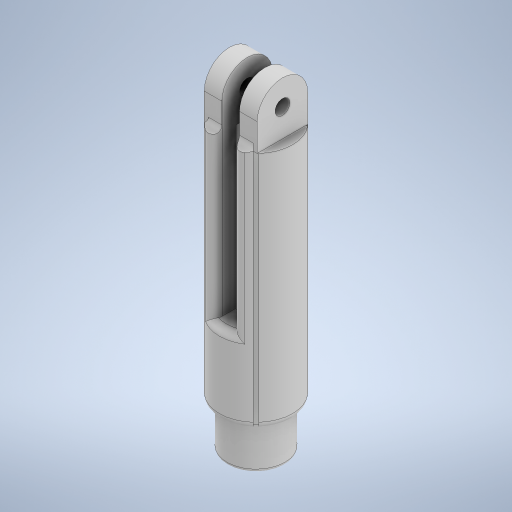
# Autodesk Inventor part: piston2
Saved by Autodesk Inventor 2024.2 (Build 282272000, 272)
## iProperties
Created: 2024-05-21
Part Number: piston2
Material: Generic
Document SubType Name: Modeling
Designer: Robin
Density: 1 g/cm^3
Appearance: Default
Author: Robin
Autodesk Inventor part; units mm, degrees
ref_plane "YZ Plane" through (0, 0, 0) normal (1, 0, 0) x (0, 1, 0)
ref_plane "XZ Plane" through (0, 0, 0) normal (0, 1, 0) x (-1, 0, 0)
ref_plane "XY Plane" through (0, 0, 0) normal (0, 0, 1) x (1, 0, 0)
sketch "Sketch1" plane through (0, 0, 0) normal (0, 1, 0) x (-1, 0, 0)
  circle A0 centre (0, 0) radius 10.375
  dimension "d0" = 20.75
  constraints: 1 centre point, 1 coincident
  measures "d0" diameter of A0
extrude "Extrusion1" add sketch "Sketch1" along normal blind 80
sketch "Sketch2" plane through (0, 80, 0) normal (0, 1, 0) x (1, 0, 0)
  line L0 (-10.375, -10.375) -> (10.375, -10.375)
  line L1 (10.375, -10.375) -> (10.375, 10.375)
  line L2 (10.375, 10.375) -> (-10.375, 10.375)
  line L3 (-10.375, 10.375) -> (-10.375, -10.375)
  circle A0 centre (0, 0) radius 10.375 projected
  line L4 (-2.5, -7.1687) -> (2.5, -7.1687)
  line L5 (2.5, -7.1687) -> (2.5, 7.1687)
  line L6 (2.5, 7.1687) -> (-2.5, 7.1687)
  line L7 (-2.5, 7.1687) -> (-2.5, -7.1687)
  line L8 (-10.375, -7.1687) -> (-7.5, -7.1687)
  line L9 (-7.5, -7.1687) -> (-7.5, 7.1687)
  line L10 (-7.5, 7.1687) -> (-10.375, 7.1687)
  line L11 (-10.375, 7.1687) -> (-10.375, -7.1687)
  line L12 (7.5, -7.1687) -> (10.375, -7.1687)
  line L13 (10.375, -7.1687) -> (10.375, 7.1687)
  line L14 (10.375, 7.1687) -> (7.5, 7.1687)
  line L15 (7.5, 7.1687) -> (7.5, -7.1687)
  line L16 (-7.5, -7.1687) -> (7.5, -7.1687)
  line L17 (-7.5, 7.1687) -> (7.5, 7.1687)
  point P0 (0, 7.1687)
  point P1 (2.5, 7.1687)
  point P2 (-2.5, 7.1687)
  dimension "d3" = 5
  dimension "d4" = 5
  dimension "d5" = 5
  constraints: 36 end point, 9 parallel, 5 horizontal, 4 perpendicular, 4 point on line, 4 tangent, 2 horizontal alignment, 2 point on circle, 1 midpoint, 1 vertical alignment
  measures "d3" distance between parallel lines of L5 L7
  measures "d4" distance between parallel lines of L9 L7
  measures "d5" distance between parallel lines of L5 L15
extrude "Extrusion2" add sketch "Sketch2" along normal blind 15 contours L9 L17 L7 L16 | L16 L5 L17 L15
sketch "Sketch4" plane through (0, 0, 0) normal (0, -1, 0) x (1, 0, 0)
  circle A0 centre (0, 0) radius 4
  line L0 (0, 0) -> (4, 0)
  line L1 (0, 0) -> (-2, -3.4641)
  line L2 (0, 0) -> (-2, 3.4641)
  circle A1 centre (0, 0) radius 10.375 projected
  line L3 (6.912, 7.7605) -> (7.7605, 6.912)
  line L4 (7.7605, 6.912) -> (6.3463, 5.4978)
  line L5 (6.3463, 5.4978) -> (5.4978, 6.3463)
  line L6 (5.4978, 6.3463) -> (6.912, 7.7605)
  line L7 (0, 0) -> (7.3362, 7.3362)
  line L8 (10.375, 0) -> (0, 0)
  point P0 (7.7482, 6.8997)
  point P1 (6.8997, 7.7482)
  dimension "d12" = 8
  dimension "d13" = 120
  dimension "d14" = 120
  dimension "d41" = 45
  dimension "d42" = 1.2
  dimension "d43" = 0.6
  dimension "d44" = 2
  constraints: 18 end point, 3 perpendicular, 3 point on circle, 2 horizontal, 1 centre point, 1 coincident, 1 parallel, 1 point on line, 4 other
  measures "d12" diameter of A0
  measures "d13" angle of L1 L0
  measures "d14" angle of L0 L2
  measures "d41" angle of L0 L7
  measures "d42" distance between parallel lines of L6 L4
  measures "d43" distance between parallel lines of L4 L7
  measures "d44" distance between parallel lines of L5 L3
extrude "Extrusion4" cut sketch "Sketch4" against normal up to surface (80 mm away) contours L2 L1 A0 | A0 L7 L2 | L1 L0 A0 | A0 L0 L7 | L7 A1 L4 L5 | L5 L6 A1 L7
sketch "Sketch9" plane through (-7.5, 80, -7.1687) normal (-1, 0, 0) x (0, 0, 1)
  circle A0 centre (7.1687, 7.8313) radius 7.1687
  line L0 (0, 15) -> (14.3375, 15) projected
  line L1 (14.3375, 0) -> (14.3375, 15) projected
  line L2 (0, 0) -> (0, 15) projected
  line L3 (0, 15) -> (14.3375, 15)
  line L4 (14.3375, 15) -> (14.3375, 7.5)
  line L5 (14.3375, 7.5) -> (0, 7.5)
  line L6 (0, 7.5) -> (0, 15)
  circle A1 centre (7.1687, 7.8313) radius 2.1
  point P0 (7.1687, -80)
  point P1 (0, 7.8313)
  point P2 (7.1687, 15)
  point P3 (14.3375, 7.8313)
  dimension "d36" = 4.2
  constraints: 8 end point, 3 tangent, 2 centre point, 2 parallel, 1 coincident, 1 horizontal, 1 midpoint, 1 perpendicular
  measures "d36" diameter of A1
extrude "Extrusion9" cut sketch "Sketch9" against normal through all contours A0 L0 L1 | A0 L2 L0 | A1 L5 | L5 A1
sketch "Sketch10" plane through (0, 0, 0) normal (0, -1, 0) x (1, 0, 0)
  circle A0 centre (0, 0) radius 4.5
  circle A1 centre (0, 0) radius 8.25
  circle A2 centre (0, 0) radius 11
  dimension "d45" = 9
  dimension "d46" = 16.5
  dimension "d47" = 22
  constraints: 3 centre point, 3 coincident
  measures "d45" diameter of A0
  measures "d46" diameter of A1
  measures "d47" diameter of A2
extrude "Extrusion10" cut sketch "Sketch10" against normal blind 12
pattern_circular "Circular Pattern2" count 4 over 360 about axis through (0, 0, 0) along (0, 1, 0) of "Extrusion4"
fillet "Fillet4" radius 2 5 edges at (-7.5, 80, 0) (-4.4101, 80, -7.1687) (4.4101, 80, -7.1687) (4.4101, 80, 7.1687) (-4.4101, 80, 7.1687)
fillet "Fillet5" radius 1 1 edges at (-8.25, 0, 0)
sketch "Sketch11" plane through (-7.5, 87.8313, 7.1687) normal (0, 0, 1) x (1, 0, 0)
  line L0 (5, -7.8313) -> (10, -7.8313)
  line L1 (10, -7.8313) -> (10, -52.8313)
  line L2 (10, -52.8313) -> (5, -52.8313)
  line L3 (5, -52.8313) -> (5, -7.8313)
  point P0 (7.5, -87.8313)
  dimension "d55" = 5
  dimension "d56" = 45
  constraints: 8 end point, 2 parallel, 1 horizontal, 1 perpendicular
  measures "d55" distance of L1.end L2.end
  measures "d56" distance of L0.end L1.end
extrude "Extrusion11" cut sketch "Sketch11" along normal through all both and the other way through all
fillet "Fillet6" radius 2 6 edges at (0, 35, 10.375) (0, 35, -10.375) (2.5, 57.5, -10.0693) (-2.5, 57.5, -10.0693) (2.5, 57.5, 10.0693) (-2.5, 57.5, 10.0693)
fillet "Fillet7" radius 2 4 edges at (0, 12, -10.375) (10.375, 12, 0) (-10.375, 12, 0) (0, 12, 10.375)
body "Solid1"
